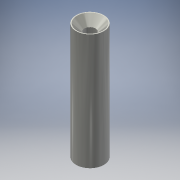
# Autodesk Inventor part: PTFE - Isolator
Saved by Autodesk Inventor 2017 (Build 210142000, 142)
## iProperties
Part Number: PTFE - Isolator
Material: Polytetrafluoroethylen
Document SubType Name: Modeling
Designer: David Merges
Density: 2.02 g/cm^3
Appearance: Glatt - Elfenbein
Author: David Merges
Autodesk Inventor part; units mm, degrees
ref_plane "YZ Plane" through (0, 0, 0) normal (1, 0, 0) x (0, 1, 0)
ref_plane "XZ Plane" through (0, 0, 0) normal (0, 1, 0) x (-1, 0, 0)
ref_plane "XY Plane" through (0, 0, 0) normal (0, 0, 1) x (1, 0, 0)
sketch "Skizze1" plane through (0, 0, 0) normal (0, 0, 1) x (1, 0, 0)
  circle A0 centre (0, 0) radius 3
  dimension "d0" = 6
  constraints: 1 centre point, 1 coincident
  measures "d0" diameter of A0
extrude "Extrusion1" add sketch "Skizze1" along normal blind 24
sketch "Skizze2" plane through (0, 0, 0) normal (0, 0, -1) x (-1, 0, 0)
  point P0 (0, 0)
hole "Bohrung1" at (0, 0, 0) direction (0, 0, 1) diameter 1.2 end through all
sketch "Skizze3" plane through (0, 0, 24) normal (0, 0, 1) x (1, 0, 0)
  point P0 (0, 0)
hole "Bohrung2" at (0, 0, 24) direction (0, 0, -1) diameter 2.4 depth 10 tip angle 118
chamfer "Fase1" distance 1.6 angle 45 1 edges at (0, 1.2, 24)
